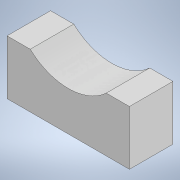
# Autodesk Inventor part: seat
Saved by Autodesk Inventor 2021 (Build 250183000, 183)
## iProperties
Created: 2021-03-31
Part Number: seat
Material: Generic
Document SubType Name: Modeling
Designer: miw14
Mass: 193838 g
Surface Area: 26179.8 cm^2
Volume: 193838 cm^3
Density: 1 g/cm^3
Appearance: Default
Author: miw14
Autodesk Inventor part; units mm, degrees
ref_plane "YZ Plane" through (0, 0, 0) normal (1, 0, 0) x (0, 1, 0)
ref_plane "XZ Plane" through (0, 0, 0) normal (0, 1, 0) x (-1, 0, 0)
ref_plane "XY Plane" through (0, 0, 0) normal (0, 0, 1) x (1, 0, 0)
sketch "Sketch1" plane through (0, 0, 0) normal (0, 0, 1) x (1, 0, 0)
  line L0 (-571.5, -254) -> (571.5, -254)
  line L1 (571.5, -254) -> (571.5, 254)
  line L2 (-571.5, 254) -> (-571.5, -254)
  line L3 (-571.5, -254) -> (571.5, 254) construction
  line L4 (571.5, -254) -> (-571.5, 254) construction
  arc A0 (-354.7976, 254) -> (354.7976, 254) centre (0, 635.113) ccw
  line L5 (571.5, 254) -> (354.7976, 254)
  line L6 (-354.7976, 254) -> (-571.5, 254)
  point P0 (0, 0)
  dimension "d0" = 1143
  dimension "d1" = 508
  dimension "d4" = 1041.4
  constraints: 14 end point, 3 parallel, 2 midpoint, 2 point on circle, 1 centre point, 1 horizontal, 1 perpendicular
  measures "d0" distance of L1.end L2.start
  measures "d1" distance of L2.start L0.start
  measures "d4" diameter of A0
extrude "Extrusion1" add sketch "Sketch1" along normal blind 406.4
sketch "Sketch4" plane through (-571.5, -254, 0) normal (0, -1, 0) x (1, 0, 0)
  line L0 (0, 406.4) -> (1143, 406.4) projected
  line L1 (571.5, 406.4) -> (571.5, 0)
  line L2 (311.1582, 406.4) -> (311.1582, 0)
  line L3 (0, 0) -> (1143, 0) projected
  line L4 (0, 0) -> (0, 406.4) projected
  line L5 (295.275, 68.2625) -> (130.175, 68.2625)
  line L6 (130.175, 68.2625) -> (130.175, 338.1375)
  line L7 (130.175, 338.1375) -> (295.275, 338.1375)
  line L8 (295.275, 338.1375) -> (295.275, 68.2625)
  line L9 (847.725, 68.2625) -> (1012.825, 68.2625)
  line L10 (1012.825, 68.2625) -> (1012.825, 338.1375)
  line L11 (1012.825, 338.1375) -> (847.725, 338.1375)
  line L12 (847.725, 338.1375) -> (847.725, 68.2625)
  dimension "d13" = 311.1582
  dimension "d14" = 165.1
  dimension "d15" = 269.875
  dimension "d16" = 68.2625
  constraints: 20 end point, 4 symmetric about line, 2 parallel, 2 point on line, 2 vertical, 1 horizontal, 1 midpoint, 1 perpendicular
  measures "d13" distance between parallel lines of L4 L2
  measures "d14" distance of L6.end L7.end
  measures "d15" distance of L5.end L6.end
  measures "d16" distance between parallel lines of L0 L7
extrude "Extrusion3" cut sketch "Sketch4" against normal blind 15.875 contours L5 L6 L7 L8 | L12 L11 L10 L9
body "Solid1"
